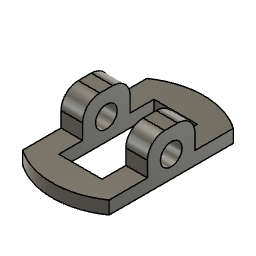
PCB Caps (Autodesk Fusion 360 design; units mm, degrees)
Autodesk Fusion 360 part; units mm, degrees
sketch "Sketch1" plane through (0, 0, 0) normal (0, 1, 0) x (1, 0, 0) in component "PCBCap"
  circle A0 centre (0, 0) radius 17.5
  dimension "d1" = 35
  constraint coincident A0.centre origin
  measures "d1" diameter of A0
extrude "Extrude1" add sketch "Sketch1" along normal blind 3 in component "PCBCap"
sketch "Sketch2" plane through (0, 3, 0) normal (0, 1, 0) x (-1, 0, 0) in component "PCBCap"
  circle A0 centre (0, 0) radius 17.5
  line L0 (10, 11) -> (10, -11)
  line L1 (-10, 11) -> (-10, -11)
  line L2 (0, 1.75) -> (0, 22.5)
  line L3 (-1.75, 0) -> (-22.5, 0)
  line L4 (10, -11) -> (5, -11)
  line L5 (5, -11) -> (5, 11)
  line L6 (5, 11) -> (10, 11)
  line L7 (10, 11) -> (10, -11)
  line L8 (-10, -11) -> (-5, -11)
  line L9 (-5, -11) -> (-5, 11)
  line L10 (-5, 11) -> (-10, 11)
  line L11 (-10, 11) -> (-10, -11)
  point P0 (10, 0)
  point P1 (-10, 0)
  dimension "d4" = 22
  dimension "d5" = 22
  dimension "d10" = 5
  dimension "d11" = 5
  dimension "d19" = 20
  constraint vertical L0
  constraint midpoint L0 P0
  constraint vertical L1
  constraint symmetric L0 L1 L2
  constraint coincident P0 L3
  constraint midpoint L1 P1
  constraint coincident L3 P1
  constraint horizontal L4
  constraint vertical L5
  constraint horizontal L6
  constraint vertical L7
  constraint horizontal L8
  constraint vertical L9
  constraint horizontal L10
  constraint vertical L11
  measures "d4" distance of L0.start L0.end
  measures "d5" distance of L1.start L1.end
  measures "d10" distance of L0.end L4.end
  measures "d11" distance of L1.end L8.end
  measures "d19" distance of L1 L7
extrude "Extrude2" add sketch "Sketch2" along normal blind 7.5 contours L0 L4 L5 L6 L7 | L1 L3 L9 L10 L11 | L1 L3 L8 L9 L11 in component "PCBCap"
sketch "Sketch3" plane through (0, 3, 0) normal (0, 1, 0) x (-1, 0, 0) in component "PCBCap"
  line L0 (-10, 11) -> (-5, 11)
  line L1 (-5, 11) -> (-5, -11)
  line L2 (-5, -11) -> (-10, -11)
  line L3 (10, -11) -> (5, -11)
  line L4 (5, -11) -> (5, 11)
  line L5 (5, 11) -> (10, 11)
  line L6 (5, 11) -> (5, -11)
  line L7 (-10, -11) -> (-10, 11)
  line L8 (10, 11) -> (10, -11)
  circle A0 centre (0, 0) radius 17.5
  line L9 (-5, 11) -> (5, 11)
  line L10 (5, 11) -> (5, -11)
  line L11 (5, -11) -> (-5, -11)
  line L12 (-5, -11) -> (-5, 11)
  line L13 (-5, 11) -> (5, -11) construction
  line L14 (5, 11) -> (-5, -11) construction
  dimension "d20" = 22
  dimension "d21" = 10
  constraint vertical L6
  constraint coincident L3.end L4.start
  constraint horizontal L9
  constraint perpendicular L9 L10
  constraint parallel L9 L11
  constraint parallel L10 L12
  constraint coincident L13 A0.centre
  constraint coincident L14 A0.centre
  constraint coincident A0.centre origin
  measures "d20" distance of L4.end L3.end
  measures "d21" distance of L3.end L1.end
extrude "Extrude3" cut sketch "Sketch3" against normal through all contours L1 L4 L6 L9 L10 L11 L12 in component "PCBCap"
sketch "Sketch2 (2)" plane through (0, 3, 0) normal (0, 1, 0) x (-1, 0, 0)
  circle A0 centre (0, 0) radius 17.5
  line L0 (-5, 11) -> (5, 11)
  line L1 (5, 11) -> (10, 11)
  line L2 (10, 11) -> (10, -11)
  line L3 (10, -11) -> (5, -11)
  line L4 (5, -11) -> (-5, -11)
  line L5 (-5, -11) -> (-10, -11)
  line L6 (-10, -11) -> (-10, 11)
  line L7 (-10, 11) -> (-5, 11)
  line L8 (10, 0) -> (20, 0)
  line L9 (20, 0) -> (20, -20)
  line L10 (20, -20) -> (10, -20)
  line L11 (10, -20) -> (10, 0)
  line L12 (10, 0) -> (20, 0)
  line L13 (20, 0) -> (20, 20)
  line L14 (20, 20) -> (10, 20)
  line L15 (10, 20) -> (10, 0)
  line L16 (-10, 0) -> (-20, 0)
  line L17 (-20, 0) -> (-20, -20)
  line L18 (-20, -20) -> (-10, -20)
  line L19 (-10, -20) -> (-10, 0)
  line L20 (-10, 0) -> (-20, 0)
  line L21 (-20, 0) -> (-20, 20)
  line L22 (-20, 20) -> (-10, 20)
  line L23 (-10, 20) -> (-10, 0)
  point P0 (10, 0)
  point P1 (-10, 0)
  dimension "d22" = 10
  dimension "d23" = 20
  dimension "d24" = 10
  dimension "d25" = 20
  dimension "d27" = 10
  dimension "d28" = 20
  dimension "d30" = 20
  constraint midpoint L2 P0
  constraint midpoint L6 P1
  constraint horizontal L8
  constraint vertical L9
  constraint horizontal L10
  constraint vertical L11
  constraint coincident P0 L8.start
  constraint horizontal L12
  constraint vertical L13
  constraint horizontal L14
  constraint vertical L15
  constraint horizontal L16
  constraint vertical L17
  constraint horizontal L18
  constraint vertical L19
  constraint coincident P1 L16.start
  constraint horizontal L20
  constraint vertical L21
  constraint horizontal L22
  constraint vertical L23
  measures "d22" distance of P0 L8.end
  measures "d23" distance of P0 L10.end
  measures "d24" distance of P0 L8.end
  measures "d25" distance of P0 L14.end
  measures "d27" distance of P1 L16.end
  measures "d28" distance of P1 L18.end
  measures "d30" distance of P1 L22.end
extrude "Extrude5" cut sketch "Sketch2 (2)" against normal through all contours A0 L2 L8 L12 L15 | A0 L2 L8 L11 L12 | A0 L6 L16 L20 L23 | A0 L6 L16 L19 L20 in component "PCBCap"
sketch "Sketch3 (2)" plane through (10, 0, 0) normal (1, 0, 0) x (0, 0, -1)
  line L0 (11, 3) -> (11, 10.5)
  line L1 (11, 10.5) -> (-11, 10.5)
  line L2 (-11, 10.5) -> (-11, 3)
  line L3 (-14.3614, 0) -> (14.3614, 0)
  circle A0 centre (0, 5) radius 2.5
  line L4 (-11, 3) -> (-14.3614, 3)
  line L5 (-14.3614, 3) -> (-14.3614, 0)
  line L6 (14.3614, 0) -> (14.3614, 3)
  line L7 (14.3614, 3) -> (11, 3)
  point P0 (-11, 5)
  point P1 (0, 5)
  dimension "d32" = 5
  constraint coincident L2 P0
  constraint coincident P1 A0.centre
  measures "d32" diameter of A0
extrude "Extrude6" cut sketch "Sketch3 (2)" against normal up to surface (20 mm away) contours A0 in component "PCBCap"
sketch "Sketch4" plane through (10, 0, 0) normal (1, 0, 0) x (0, 0, -1)
  circle A0 centre (0, 5) radius 2.5
  line L0 (11, 3) -> (11, 10.5)
  line L1 (11, 10.5) -> (-11, 10.5)
  line L2 (-11, 10.5) -> (-11, 3)
  line L3 (-14.3614, 0) -> (14.3614, 0)
  line L4 (-11, 5) -> (0, 5)
  line L5 (0, 5) -> (11, 5)
  line L6 (-5.5, 5) -> (-11, 5)
  line L7 (-11, 5) -> (-11, 10.5)
  line L8 (-11, 10.5) -> (-5.5, 10.5)
  line L9 (-5.5, 10.5) -> (-5.5, 5)
  line L10 (-5.5, 5) -> (-11, 5)
  line L11 (-11, 5) -> (-11, 3)
  line L12 (-11, 3) -> (-5.5, 3)
  line L13 (-5.5, 3) -> (-5.5, 5)
  line L14 (5.5, 5) -> (11, 5)
  line L15 (11, 5) -> (11, 10.5)
  line L16 (11, 10.5) -> (5.5, 10.5)
  line L17 (5.5, 10.5) -> (5.5, 5)
  line L18 (5.5, 5) -> (11, 5)
  line L19 (11, 5) -> (11, 3)
  line L20 (11, 3) -> (5.5, 3)
  line L21 (5.5, 3) -> (5.5, 5)
  line L22 (-11, 3) -> (-14.3614, 3)
  line L23 (-14.3614, 3) -> (-14.3614, 0)
  line L24 (14.3614, 0) -> (14.3614, 3)
  line L25 (14.3614, 3) -> (11, 3)
  point P0 (0, 5)
  point P1 (-11, 5)
  point P2 (11, 5)
  point P3 (-5.5, 5)
  point P4 (5.5, 5)
  constraint coincident P0 A0.centre
  constraint coincident L2 P1
  constraint coincident L0 P2
  constraint coincident P1 L4.start
  constraint perpendicular L2 L4
  constraint midpoint L4 P3
  constraint coincident P2 L5.end
  constraint perpendicular L0 L5
  constraint midpoint P4 L5
  constraint horizontal L6
  constraint vertical L7
  constraint horizontal L8
  constraint vertical L9
  constraint coincident L1.end L2.start
  constraint coincident P3 L6.start
  constraint horizontal L10
  constraint vertical L11
  constraint horizontal L12
  constraint vertical L13
  constraint coincident L2.end L11.end
  constraint horizontal L14
  constraint vertical L15
  constraint horizontal L16
  constraint vertical L17
  constraint coincident L0.end L1.start
  constraint coincident P4 L14.start
  constraint horizontal L18
  constraint vertical L19
  constraint horizontal L20
  constraint vertical L21
  constraint coincident L0.start L19.end
extrude "Extrude7" cut sketch "Sketch4" against normal through all contours L0 L1 L5 L14 L15 L16 L17 L18 | L0 L5 L14 L18 L19 L20 L21 | L2 L4 L6 L10 L11 L12 L13 | L1 L2 L4 L6 L7 L8 L9 L10 in component "PCBCap"
fillet "Fillet1" radius 4 4 edges at (7.5, 10.5, 5.5) (7.5, 10.5, -5.5) (-7.5, 10.5, 5.5) (-7.5, 10.5, -5.5) in component "PCBCap"
sketch "Sketch1 (2)" plane through (0, 3, 0) normal (0, 1, 0) x (-1, 0, 0)
  line L0 (10, 5.5) -> (23.3893, 5.5)
  line L1 (23.3893, 5.5) -> (23.3893, -16.5)
  line L2 (23.3893, -16.5) -> (10, -16.5)
  line L3 (10, -16.5) -> (10, 5.5)
  line L4 (-13.6107, -11) -> (-19, -11)
  line L5 (-19, -11) -> (-19, 11)
  line L6 (-19, 11) -> (-13.6107, 11)
  line L7 (-13.6107, 11) -> (-13.6107, -11)
  line L8 (10, 5.5) -> (10, 14.3614)
  line L9 (-5, 11) -> (5, 11)
  line L10 (5, -11) -> (-5, -11)
  line L11 (-10, 14.3614) -> (-10, 5.5)
  line L12 (-10, 5.5) -> (-5, 5.5)
  line L13 (-5, 5.5) -> (-5, 11)
  line L14 (5, 11) -> (5, 5.5)
  line L15 (5, 5.5) -> (10, 5.5)
  arc A0 (10, 14.3614) -> (-10, 14.3614) centre (0, 0) ccw
  line L16 (-10, -5.5) -> (-10, -14.3614)
  arc A1 (-10, -14.3614) -> (10, -14.3614) centre (0, 0) ccw
  line L17 (10, -14.3614) -> (10, -5.5)
  line L18 (10, -5.5) -> (5, -5.5)
  line L19 (5, -5.5) -> (5, -11)
  line L20 (-5, -11) -> (-5, -5.5)
  line L21 (-5, -5.5) -> (-10, -5.5)
  constraint horizontal L0
  constraint vertical L1
  constraint horizontal L2
  constraint vertical L3
  constraint coincident L0.start L3.end
  constraint horizontal L4
  constraint vertical L5
  constraint horizontal L6
  constraint vertical L7
extrude "Extrude4" cut sketch "Sketch1 (2)" against normal through all contours L0 L1 L2 L3 L17 | L4 L5 L6 L7 in component "PCBCap"
component "PCBCap" placed x (1, 0, 0) y (0, 1, 0) z (0, 0, 1) at (0, 0, 0)
equation "d4 = PCBWidth + 2 * ( PCBWidthTolerance )"
equation "d5 = PCBWidth + 2 * ( PCBWidthTolerance )"
equation "PCBWidth = 20 mm" comment "Width of the PCB"
equation "PCBWidthTolerance = 1 mm" comment "Additional Width for PCB"
equation "PCBWallThickness = 5 mm" comment "Thickness of PCB Wall"
equation "d10 = PCBWallThickness"
equation "d11 = PCBWallThickness"
equation "PCBWallSpread = 20 mm" comment "Distance between the two PCB Walls"
equation "PCBWallLength = 7.5 mm" comment "Length of the PCB Wall for screwing in"
equation "d19 = PCBWallSpread"
equation "d20 = PCBWidth + 2 * PCBWidthTolerance"
equation "d21 = PCBWallSpread - 2 * ( PCBWallThickness )"
equation "d23 = PCBWidth"
equation "d25 = PCBWidth"
equation "d28 = PCBWidth"
equation "d30 = PCBWidth"
